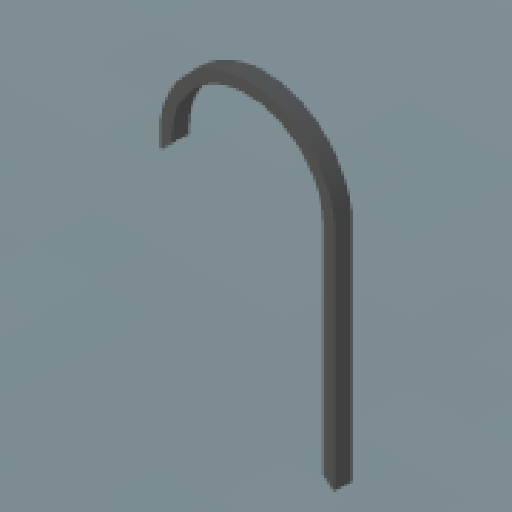
# Autodesk Inventor part: Drag Chain Dummy
Saved by Autodesk Inventor 2023.2 (Build 272271000, 271)
## iProperties
Created: 2023-02-07
Part Number: Drag Chain Dummy
Material: ABS Plastic
Document SubType Name: Modeling
Designer: remop
Density: 1.06 g/cm^3
Appearance: Gray
Author: remop
Autodesk Inventor part; units mm, degrees
ref_plane "YZ Plane" through (0, 0, 0) normal (1, 0, 0) x (0, 1, 0)
ref_plane "XZ Plane" through (0, 0, 0) normal (0, 1, 0) x (-1, 0, 0)
ref_plane "XY Plane" through (0, 0, 0) normal (0, 0, 1) x (1, 0, 0)
sketch "Sketch1" plane through (0, 0, 0) normal (0, 0, 1) x (1, 0, 0)
  line L0 (2, 0) -> (2, -17.9997) projected
  line L1 (226, 217) -> (226, -317) projected
  arc A0 (226, 0) -> (2, 0) centre (114, 0) ccw
  line L2 (2, -17.9997) -> (5, -17.9997)
  line L3 (5, -17.9997) -> (17, -5.9997)
  line L4 (17, -5.9997) -> (17, 0)
  line L5 (211, 0) -> (211, -275)
  line L6 (211, -275) -> (223, -287)
  line L7 (223, -287) -> (226, -287)
  arc A1 (211, 0) -> (17, 0) centre (114, 0) ccw
  point P0 (0, 0)
  point P1 (114, 112)
  point P2 (114, 97)
  dimension "d0" = 15
  dimension "d1" = 45
  dimension "d2" = 3
  dimension "d3" = 15
  dimension "d4" = 45
  dimension "d5" = 30
  dimension "d6" = 15
  constraints: 12 end point, 6 point on circle, 4 tangent, 2 centre point, 2 parallel, 2 perpendicular, 2 point on line, 1 horizontal
  measures "d0" distance between parallel lines of L0 L4
  measures "d1" angle of L4 L3
  measures "d2" distance of L0.end L2.end
  measures "d3" distance between parallel lines of L1 L5
  measures "d4" angle of L6 L5
  measures "d5" distance from line of L1.end L7
  measures "d6" distance of point (114, 112) point (114, 97)
extrude "Extrusion1" add sketch "Sketch1" against normal blind 22
equation "\"d3\" = d0"
equation "\"d4\" = d1"
equation "\"d6\" = d0"
body "Solid1"
